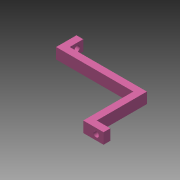
# Autodesk Inventor part: Part13
Saved by Autodesk Inventor 2015 (Build 190159000, 159)
## iProperties
Created: 2015-07-08
Part Number: Part13
Material: ABS Plastic
Document SubType Name: Modeling
Designer: eefred
Density: 1.06 g/cm^3
Appearance: Pink
Author: eefred
Autodesk Inventor part; units mm, degrees
ref_plane "YZ Plane" through (0, 0, 0) normal (1, 0, 0) x (0, 1, 0)
ref_plane "XZ Plane" through (0, 0, 0) normal (0, 1, 0) x (-1, 0, 0)
ref_plane "XY Plane" through (0, 0, 0) normal (0, 0, 1) x (1, 0, 0)
sketch "Sketch1" plane through (0, 0, 0) normal (0, 0, 1) x (1, 0, 0)
  line L0 (0, 37) -> (0, 52)
  line L1 (0, 52) -> (5, 52)
  line L2 (5, 52) -> (5, 42)
  line L3 (5, 42) -> (62, 42)
  line L4 (62, 42) -> (62, 5)
  line L5 (62, 5) -> (72, 5)
  line L6 (72, 5) -> (72, 0)
  line L7 (72, 0) -> (57, 0)
  line L8 (57, 0) -> (57, 37)
  line L9 (57, 37) -> (0, 37)
  point P0 (0, 0)
  dimension "d0" = 37
  dimension "d1" = 57
  dimension "d2" = 5
  dimension "d3" = 5
  dimension "d4" = 5
  dimension "d5" = 5
  dimension "d6" = 15
  dimension "d7" = 15
  constraints: 20 end point, 7 perpendicular, 2 vertical, 1 parallel
  measures "d0" distance of L7.end L8.end
  measures "d1" distance of L8.end L0.start
  measures "d2" distance of L0.end L1.end
  measures "d3" distance of L5.end L6.end
  measures "d4" distance between parallel lines of L9 L3
  measures "d5" distance between parallel lines of L4 L8
  measures "d6" distance of L6.end L7.end
  measures "d7" distance of L0.start L0.end
extrude "Extrusion1" add sketch "Sketch1" along normal blind 8
sketch "Sketch2" plane through (0, 37, 0) normal (-1, 0, 0) x (0, 0, 1)
  circle A0 centre (4, 10.5) radius 2
  line L0 (0, 15) -> (8, 15) projected
  point P0 (0, -37)
  point P1 (4, 15)
  dimension "d10" = 4
  dimension "d11" = 4.5
  constraints: 1 centre point, 1 midpoint, 1 vertical alignment
  measures "d10" diameter of A0
  measures "d11" distance from line of L0 A0.centre
extrude "Extrusion2" cut sketch "Sketch2" against normal up to next
sketch "Sketch3" plane through (57, 0, 0) normal (0, -1, 0) x (1, 0, 0)
  circle A0 centre (9.5, 4) radius 2
  line L0 (15, 0) -> (15, 8) projected
  point P0 (-57, 0)
  point P1 (15, 4)
  dimension "d14" = 4
  dimension "d15" = 5.5
  constraints: 1 centre point, 1 horizontal alignment, 1 midpoint
  measures "d14" diameter of A0
  measures "d15" distance from line of A0.centre L0
extrude "Extrusion3" cut sketch "Sketch3" against normal up to next
equation "\"d3\" = d2"
equation "\"d4\" = d2"
equation "\"d5\" = d2"
body "Solid1"
